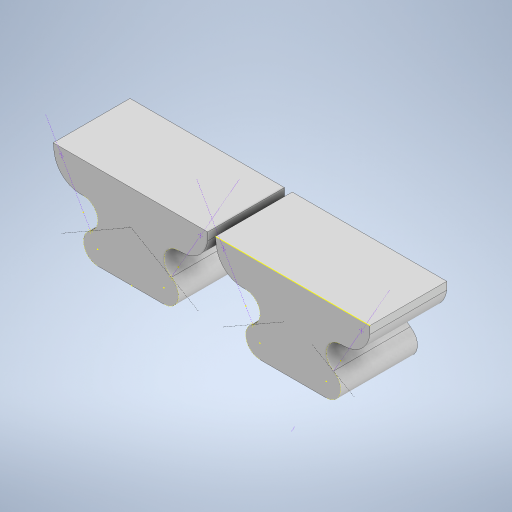
# Autodesk Inventor part: Zipperteethv4
Saved by Autodesk Inventor 2023.1 (Build 271208000, 208)
## iProperties
Created: 2022-10-04
Part Number: Zipperteethv4
Material: Generic
Document SubType Name: Modeling
Designer: Grimm
Density: 1 g/cm^3
Appearance: Default
Author: Grimm
Autodesk Inventor part; units mm, degrees
ref_plane "YZ Plane" through (0, 0, 0) normal (1, 0, 0) x (0, 1, 0)
ref_plane "XZ Plane" through (0, 0, 0) normal (0, 1, 0) x (-1, 0, 0)
ref_plane "XY Plane" through (0, 0, 0) normal (0, 0, 1) x (1, 0, 0)
sketch "Sketch1" plane through (0, 0, 0) normal (0, 0, 1) x (1, 0, 0)
  line L0 (0, 0) -> (21, 0)
  line L1 (21, 0) -> (21, 11)
  line L2 (21, 11) -> (0, 11)
  line L3 (0, 11) -> (0, 0)
  dimension "d0" = 21
  dimension "d1" = 11
  constraints: 8 end point, 2 parallel, 1 horizontal, 1 perpendicular
  measures "d0" distance of L2.end L1.end
  measures "d1" distance of L0.end L1.end
extrude "Extrusion1" add sketch "Sketch1" along normal blind 10
sketch "Sketch2" plane through (0, 0, 10) normal (0, 0, 1) x (1, 0, 0)
  line L0 (0, 0) -> (21, 0) projected
  arc A0 (4.3181, 0) -> (5.25, 3.5) centre (4.3181, 1.8741) ccw
  arc A1 (6.1819, 7) -> (5.25, 3.5) centre (6.1819, 5.1259) ccw
  arc A2 (15.75, 3.5) -> (16.6819, 0) centre (16.6819, 1.8741) ccw
  arc A3 (15.75, 3.5) -> (14.8181, 7) centre (14.8181, 5.1259) ccw
  line L1 (6.1819, 7) -> (14.8181, 7)
  line L2 (21, 11) -> (0, 11) projected
  line L3 (4.3181, 1.8741) -> (6.1819, 5.1259) construction
  line L4 (16.6819, 1.8741) -> (14.8181, 5.1259) construction
  line L5 (0, 11) -> (0, 0) construction
  line L6 (21, 0) -> (21, 11) construction
  point P0 (10.5, 7)
  point P1 (15.75, 3.5)
  dimension "d7" = 10.5
  dimension "d9" = 7
  dimension "d13" = 10.5
  constraints: 8 point on circle, 6 end point, 6 tangent, 4 centre point, 3 equal radius, 3 midpoint, 2 point on line, 1 horizontal
  measures "d7" distance of A2.start A0.end
  measures "d9" distance between parallel lines of L0 L1
  measures "d13" distance from line of L5 point (10.5, 7)
extrude "Extrusion2" cut sketch "Sketch2" against normal through all
sketch "Sketch3" plane through (0, 0, 10) normal (0, 0, 1) x (1, 0, 0)
  line L0 (21, 11) -> (0, 11) projected
  line L1 (14.8181, 7) -> (6.1819, 7) projected
  arc A0 (6.6147, 7) -> (10, 10) centre (6.6147, 10.41) ccw
  arc A1 (11, 10) -> (14.3853, 7) centre (14.3853, 10.41) ccw
  line L2 (10, 10) -> (11, 10)
  line L3 (6.1819, 7) -> (14.8181, 7) projected
  line L4 (10.5, 10) -> (10.5, 11) construction
  point P0 (0, 0)
  dimension "d15" = 1
  dimension "d16" = 1
  constraints: 4 end point, 4 point on circle, 2 centre point, 2 midpoint, 2 point on line, 2 tangent, 1 equal radius, 1 vertical
  measures "d15" distance of L2.start L2.end
  measures "d16" distance between parallel lines of L0 L2
extrude "Extrusion3" cut sketch "Sketch3" against normal through all
pattern_linear "Rectangular Pattern1" count 6 spacing 21 along (1, 0, 0)
sketch "Sketch4" plane through (0, 0, 10) normal (0, 0, 1) x (1, 0, 0)
  line L0 (115, 10) -> (116, 10) projected
  line L1 (115, 10) -> (115, 11)
  line L2 (126, 11) -> (0, 11) projected
  line L3 (121.6819, 0) -> (126, 0) projected
  line L4 (121.6819, 0) -> (126, 0)
  line L5 (126, 0) -> (126, 11)
  line L6 (126, 0) -> (126, 11) projected
  line L7 (126, 11) -> (115, 11)
  arc A0 (116, 10) -> (119.3853, 7) centre (119.3853, 10.41) ccw projected
  line L8 (115, 10) -> (116, 10)
  line L9 (119.3853, 7) -> (119.8181, 7) projected
  arc A1 (116, 10) -> (119.3853, 7) centre (119.3853, 10.41) ccw
  arc A2 (120.75, 3.5) -> (119.8181, 7) centre (119.8181, 5.1259) ccw projected
  line L10 (119.3853, 7) -> (119.8181, 7)
  arc A3 (120.75, 3.5) -> (119.8181, 7) centre (119.8181, 5.1259) ccw
  arc A4 (120.75, 3.5) -> (121.6819, 0) centre (121.6819, 1.8741) ccw projected
  arc A5 (120.75, 3.5) -> (121.6819, 0) centre (121.6819, 1.8741) ccw
  line L11 (32, 10) -> (31, 10) projected
  line L12 (31, 10) -> (31, 11)
  line L13 (31, 10) -> (31, 0)
  line L14 (31, 0) -> (126, 0)
  line L15 (126, 11) -> (31, 11)
  arc A6 (11, 10) -> (14.3853, 7) centre (14.3853, 10.41) ccw projected
  line L16 (11, 10) -> (10.8789, 11)
  line L17 (10.8789, 11) -> (0, 11)
  line L18 (0, 11) -> (0, 0)
  line L19 (0, 0) -> (11, 0)
  line L20 (11, 0) -> (11, 10)
  point P0 (11, 11)
  constraints: 30 end point, 7 point on circle, 6 perpendicular, 6 point on line, 6 tangent, 3 centre point, 3 horizontal, 1 collinear, 1 vertical
extrude "Extrusion4" cut sketch "Sketch4" against normal through all
pattern_linear "Rectangular Pattern2" count 2 spacing 21.121 along (-1, 0, 0)
sketch "Sketch5" plane through (0, 0, 10) normal (0, 0, 1) x (1, 0, 0)
  line L0 (31, 11) -> (10.8789, 11) projected
  line L1 (15.75, 3.5) -> (11.9442, 10.1401) construction
  arc A0 (15.75, 3.5) -> (16.6819, 0) centre (16.6819, 1.8741) ccw construction
  line L2 (11.7707, 1.2193) -> (15.75, 3.5) construction
  arc A1 (15.75, 3.5) -> (14.8181, 7) centre (14.8181, 5.1259) ccw construction
  line L3 (15.75, 3.5) -> (19.849, 5.8494) construction
  arc A2 (25.3181, 0) -> (26.25, 3.5) centre (25.3181, 1.8741) ccw construction
  line L4 (26.25, 3.5) -> (29.888, 9.8474) construction
  line L5 (23.4673, 5.0949) -> (26.25, 3.5) construction
  line L6 (26.25, 3.5) -> (28.9514, 1.9517) construction
  arc A3 (25.3181, 0) -> (26.25, 3.5) centre (25.3181, 1.8741) ccw construction
  line L7 (11.9442, 10.1401) -> (8.4243, 16.2814) construction
  line L8 (29.888, 9.8474) -> (33.5756, 16.2813) construction
  line L9 (21.2593, -5.2075) -> (20.7407, -6.1122) construction
  line L10 (-11.2522, 13.7611) -> (-5.371, 3.5) construction
  line L11 (-9.2047, 1.3027) -> (-5.371, 3.5) construction
  line L12 (-5.371, 3.5) -> (-0.1045, 6.5185) construction
  line L13 (5.129, 3.5) -> (8.7239, 1.4396) construction
  line L14 (5.129, 3.5) -> (-0.283, 6.6019) construction
  arc A4 (4.1971, 0) -> (5.129, 3.5) centre (4.1971, 1.8741) ccw construction
  arc A5 (-5.371, 3.5) -> (-6.3029, 7) centre (-6.3029, 5.1259) ccw construction
  arc A6 (-5.371, 3.5) -> (-4.4391, 0) centre (-4.4391, 1.8741) ccw construction
  arc A7 (6.0609, 7) -> (5.129, 3.5) centre (6.0609, 5.1259) ccw construction
  arc A8 (4.1971, 0) -> (5.129, 3.5) centre (4.1971, 1.8741) ccw construction
  line L15 (5.129, 3.5) -> (13.9975, 18.9732) construction
  arc A9 (15.75, 3.5) -> (16.6819, 0) centre (16.6819, 1.8741) ccw construction
  arc A10 (15.75, 3.5) -> (14.8181, 7) centre (14.8181, 5.1259) ccw construction
  arc A11 (27.1819, 7) -> (26.25, 3.5) centre (27.1819, 5.1259) ccw construction
  point P0 (0, 0)
  point P1 (8.9348, 10.1401)
  point P2 (-9.1768, 10.1401)
  constraints: 30 end point, 11 tangent, 5 point on line, 4 perpendicular, 2 coincident, 1 collinear
body "Solid1"
